Autodesk Fusion 360 part; units mm, degrees
(part 3 of 4)
sketch "Sketch28" plane through (0, 0, 0.5) normal (0, 0, 1) x (-1, 0, 0)
  circle A0 centre (52.75, -70) radius 2
  circle A1 centre (59.75, -70) radius 2
  circle A2 centre (45.75, -70) radius 2
  circle A3 centre (66.75, -70) radius 2
  circle A4 centre (38.75, -70) radius 2
  circle A5 centre (-106, -68.6442) radius 1.5
  circle A6 centre (-99, -68.6442) radius 1.5
  circle A7 centre (-92, -68.6442) radius 1.5
  circle A8 centre (-96.9706, 17.0711) radius 4.5
  line L0 (-64.4557, -59.7611) -> (-70.6729, -68.3891)
  line L1 (-70.6729, -68.3891) -> (-87.8309, -68.3891)
  line L2 (-87.8309, -68.3891) -> (-87.8309, -48.5956)
  line L3 (-87.8309, -48.5956) -> (-64.4557, -59.7611)
  line L4 (-5, -35.2698) -> (-5.0893, -45.8041)
  line L5 (-5.0893, -45.8041) -> (-79.6826, -45.1714)
  line L6 (-79.6826, -45.1714) -> (-64.4557, -34.7655)
  line L7 (-64.4557, -34.7655) -> (-5, -35.2698)
  line L8 (35, -50.5455) -> (35, -5)
  line L9 (35, -5) -> (80, 5)
  line L10 (80, 5) -> (99.8546, 5)
  line L11 (99.8546, 5) -> (35, -50.5455)
  line L12 (-49.2268, -20.3093) -> (-41.9977, -4.5677)
  line L13 (-41.9977, -4.5677) -> (-17.7598, -4.7733)
  line L14 (-17.7598, -4.7733) -> (-5, -9.2623)
  line L15 (-5, -9.2623) -> (-5.0969, -20.6836)
  line L16 (-5.0969, -20.6836) -> (-49.2268, -20.3093)
  line L17 (115, -15.9161) -> (115, -61.1347)
  line L18 (115, -61.1347) -> (67.4273, -61.1347)
  line L19 (67.4273, -61.1347) -> (115, -15.9161)
  circle A9 centre (-183, -68.6442) radius 1.5
  circle A10 centre (-155, -68.6442) radius 1.5
  circle A11 centre (-127, -68.6442) radius 1.5
  circle A12 centre (-120, -68.6442) radius 1.5
  circle A13 centre (-148, -68.6442) radius 1.5
  circle A14 centre (-176, -68.6442) radius 1.5
  circle A15 centre (-162, -68.6442) radius 1.5
  circle A16 centre (-134, -68.6442) radius 1.5
  circle A17 centre (-113, -68.6442) radius 1.5
  circle A18 centre (-141, -68.6442) radius 1.5
  circle A19 centre (-169, -68.6442) radius 1.5
  circle A20 centre (-181.8234, 101.9239) radius 4.5
  circle A21 centre (-125.2548, 45.3553) radius 4.5
  circle A22 centre (-139.397, 59.4975) radius 4.5
  circle A23 centre (-167.6812, 87.7817) radius 4.5
  circle A24 centre (-111.1127, 31.2132) radius 4.5
  circle A25 centre (-153.5391, 73.6396) radius 4.5
  circle A26 centre (87.75, -70) radius 2
  circle A27 centre (108.75, -70) radius 2
  circle A28 centre (80.75, -70) radius 2
  circle A29 centre (94.75, -70) radius 2
  circle A30 centre (101.75, -70) radius 2
  circle A31 centre (73.75, -70) radius 2
  circle A32 centre (101.6789, -8.3211) radius 5
  circle A33 centre (108.75, -80) radius 2
  circle A34 centre (86.25, -80) radius 2
  circle A35 centre (63.75, -80) radius 2
  circle A36 centre (41.25, -77.5) radius 2
  circle A37 centre (73.3947, -36.6053) radius 5
  circle A38 centre (87.5368, -22.4632) radius 5
  line L20 (120, -80) -> (120, 10)
  line L21 (120, 10) -> (75, 10)
  line L22 (75, 10) -> (30, 0)
  line L23 (30, 0) -> (0, 0)
  line L24 (0, 0) -> (-45, 10)
  line L25 (-45, 10) -> (-75.7574, 10)
  line L26 (-75.7574, 10) -> (-181.8234, 116.066)
  line L27 (-181.8234, 116.066) -> (-195.9655, 101.9239)
  line L28 (-195.9655, 101.9239) -> (-90, -4.0416)
  line L29 (-90, -4.0416) -> (-90, -62.2885)
  line L30 (-90, -62.2885) -> (-190, -62.2885)
  line L31 (-190, -62.2885) -> (-190, -75)
  line L32 (-190, -75) -> (-90, -75)
  line L33 (-90, -75) -> (-90, -80)
  line L34 (-90, -80) -> (-22.5, -80)
  line L35 (-22.5, -80) -> (0, -75)
  line L36 (0, -75) -> (30, -75)
  line L37 (30, -75) -> (37.3453, -76.6323)
  line L38 (37.3453, -76.6323) -> (37.3453, -83.3677)
  line L39 (37.3453, -83.3677) -> (45.1547, -83.3677)
  line L40 (45.1547, -83.3677) -> (45.1547, -78.3677)
  line L41 (45.1547, -78.3677) -> (52.5, -80)
  line L42 (52.5, -80) -> (59.75, -80)
  line L43 (59.75, -80) -> (59.75, -85)
  line L44 (59.75, -85) -> (67.75, -85)
  line L45 (67.75, -85) -> (67.75, -80)
  line L46 (67.75, -80) -> (82.25, -80)
  line L47 (82.25, -80) -> (82.25, -85)
  line L48 (82.25, -85) -> (90.25, -85)
  line L49 (90.25, -85) -> (90.25, -80)
  line L50 (90.25, -80) -> (104.75, -80)
  line L51 (104.75, -80) -> (104.75, -85)
  line L52 (104.75, -85) -> (112.75, -85)
  line L53 (112.75, -85) -> (112.75, -80)
  line L54 (112.75, -80) -> (120, -80)
  line L55 (-14.25, -68.5) -> (-8.25, -68.5)
  line L56 (-8.25, -68.5) -> (-8.25, -71.5)
  line L57 (-8.25, -71.5) -> (-14.25, -71.5)
  line L58 (-14.25, -71.5) -> (-14.25, -68.5)
  line L59 (-72.1594, -47.0213) -> (-67.271, -50.5004)
  line L60 (-67.271, -50.5004) -> (-69.0348, -52.9787)
  line L61 (-69.0348, -52.9787) -> (-73.9232, -49.4996)
  line L62 (-73.9232, -49.4996) -> (-72.1594, -47.0213)
  line L63 (-58.1594, -27.0213) -> (-53.271, -30.5004)
  line L64 (-53.271, -30.5004) -> (-55.0348, -32.9787)
  line L65 (-55.0348, -32.9787) -> (-59.9232, -29.4996)
  line L66 (-59.9232, -29.4996) -> (-58.1594, -27.0213)
  line L67 (-10.5728, -3.1023) -> (-4.573, -3.1532)
  line L68 (-4.573, -3.1532) -> (-4.5984, -6.1531)
  line L69 (-4.5984, -6.1531) -> (-10.5982, -6.1022)
  line L70 (-10.5982, -6.1022) -> (-10.5728, -3.1023)
  line L71 (-67.8203, 7.9003) -> (-65.8203, 7.9003)
  line L72 (-65.8203, 7.9003) -> (-65.8203, 5.9003)
  line L73 (-65.8203, 5.9003) -> (-67.8203, 5.9003)
  line L74 (-67.8203, 5.9003) -> (-67.8203, 7.9003)
  line L75 (-76.9306, -16.181) -> (-75.5164, -17.5952)
  line L76 (-75.5164, -17.5952) -> (-76.9306, -19.0095)
  line L77 (-76.9306, -19.0095) -> (-78.3448, -17.5952)
  line L78 (-78.3448, -17.5952) -> (-76.9306, -16.181)
  line L79 (-87.8309, -27.9541) -> (-85.8309, -27.9541)
  line L80 (-85.8309, -27.9541) -> (-85.8309, -29.9541)
  line L81 (-85.8309, -29.9541) -> (-87.8309, -29.9541)
  line L82 (-87.8309, -29.9541) -> (-87.8309, -27.9541)
  line L83 (-66.3319, -10.7541) -> (-65.4866, -8.9415)
  line L84 (-65.4866, -8.9415) -> (-63.674, -9.7867)
  line L85 (-63.674, -9.7867) -> (-64.5193, -11.5994)
  line L86 (-64.5193, -11.5994) -> (-66.3319, -10.7541)
  line L87 (-42.179, 1.1199) -> (-36.1792, 1.0739)
  line L88 (-36.1792, 1.0739) -> (-36.2025, -1.9678)
  line L89 (-36.2025, -1.9678) -> (-42.2023, -1.9219)
  line L90 (-42.2023, -1.9219) -> (-42.179, 1.1199)
  line L91 (-10.5728, -25.1023) -> (-4.573, -25.1532)
  line L92 (-4.573, -25.1532) -> (-4.5984, -28.1531)
  line L93 (-4.5984, -28.1531) -> (-10.5982, -28.1022)
  line L94 (-10.5982, -28.1022) -> (-10.5728, -25.1023)
  line L95 (-11.9719, -47.9791) -> (-6.0721, -49.071)
  line L96 (-6.0721, -49.071) -> (-6.6181, -52.0209)
  line L97 (-6.6181, -52.0209) -> (-12.5179, -50.929)
  line L98 (-12.5179, -50.929) -> (-11.9719, -47.9791)
  line L99 (-81.75, -71.5367) -> (-75.75, -71.5367)
  line L100 (-75.75, -71.5367) -> (-75.75, -74.5367)
  line L101 (-75.75, -74.5367) -> (-81.75, -74.5367)
  line L102 (-81.75, -74.5367) -> (-81.75, -71.5367)
  line L103 (-36.75, -71.5367) -> (-30.75, -71.5367)
  line L104 (-30.75, -71.5367) -> (-30.75, -74.5367)
  line L105 (-30.75, -74.5367) -> (-36.75, -74.5367)
  line L106 (-36.75, -74.5367) -> (-36.75, -71.5367)
  line L107 (-50.7607, -47.5524) -> (-45.1333, -49.6339)
  line L108 (-45.1333, -49.6339) -> (-46.174, -52.4476)
  line L109 (-46.174, -52.4476) -> (-51.8014, -50.3661)
  line L110 (-51.8014, -50.3661) -> (-50.7607, -47.5524)
  line L111 (-43.7607, -25.5524) -> (-38.1333, -27.6339)
  line L112 (-38.1333, -27.6339) -> (-39.174, -30.4476)
  line L113 (-39.174, -30.4476) -> (-44.8014, -28.3661)
  line L114 (-44.8014, -28.3661) -> (-43.7607, -25.5524)
  line L115 (-24.686, 0.859) -> (-18.6861, 0.8794)
  line L116 (-18.6861, 0.8794) -> (-18.6759, -2.1206)
  line L117 (-18.6759, -2.1206) -> (-24.6759, -2.141)
  line L118 (-24.6759, -2.141) -> (-24.686, 0.859)
  line L119 (-62.1634, 5.9003) -> (-62.1634, 7.9003)
  line L120 (-62.1634, 7.9003) -> (-60.1634, 7.9003)
  line L121 (-60.1634, 7.9003) -> (-60.1634, 5.9003)
  line L122 (-60.1634, 5.9003) -> (-62.1634, 5.9003)
  line L123 (-72.9306, -20.181) -> (-71.5164, -21.5952)
  line L124 (-71.5164, -21.5952) -> (-72.9306, -23.0095)
  line L125 (-72.9306, -23.0095) -> (-74.3448, -21.5952)
  line L126 (-74.3448, -21.5952) -> (-72.9306, -20.181)
  line L127 (-87.8309, -19.8881) -> (-85.8309, -19.8881)
  line L128 (-85.8309, -19.8881) -> (-85.8309, -21.8881)
  line L129 (-85.8309, -21.8881) -> (-87.8309, -21.8881)
  line L130 (-87.8309, -21.8881) -> (-87.8309, -19.8881)
  line L131 (-70.6135, -6.5508) -> (-68.8009, -7.396)
  line L132 (-68.8009, -7.396) -> (-69.6461, -9.2087)
  line L133 (-69.6461, -9.2087) -> (-71.4587, -8.3634)
  line L134 (-71.4587, -8.3634) -> (-70.6135, -6.5508)
  line L135 (-35.0324, 0.9507) -> (-29.0325, 0.9195)
  line L136 (-29.0325, 0.9195) -> (-29.0481, -2.0804)
  line L137 (-29.0481, -2.0804) -> (-35.048, -2.0492)
  line L138 (-35.048, -2.0492) -> (-35.0324, 0.9507)
  line L139 (-28.0908, -25.011) -> (-22.1784, -26.0328)
  line L140 (-22.1784, -26.0328) -> (-22.6893, -28.989)
  line L141 (-22.6893, -28.989) -> (-28.6017, -27.9672)
  line L142 (-28.6017, -27.9672) -> (-28.0908, -25.011)
  line L143 (-26.6893, -51.989) -> (-32.6017, -50.9672)
  line L144 (-32.6017, -50.9672) -> (-32.0908, -48.011)
  line L145 (-32.0908, -48.011) -> (-26.1784, -49.0328)
  line L146 (-26.1784, -49.0328) -> (-26.6893, -51.989)
  line L147 (-59.25, -71.5367) -> (-53.25, -71.5367)
  line L148 (-53.25, -71.5367) -> (-53.25, -74.5367)
  line L149 (-53.25, -74.5367) -> (-59.25, -74.5367)
  line L150 (-59.25, -74.5367) -> (-59.25, -71.5367)
  line L151 (-45, -57) -> (-5, -57)
  line L152 (-5, -57) -> (-5, -60)
  line L153 (-5, -60) -> (-45, -60)
  arc A39 (-45, -60) -> (-66.3234, -75) centre (-45, -82.6562) ccw
  line L154 (-66.3234, -75) -> (-69.4872, -75)
  arc A40 (-45, -57) -> (-69.4872, -75) centre (-45, -82.6562) ccw
  line L155 (0, -5) -> (30, -5)
  line L156 (30, -5) -> (30, -70)
  line L157 (30, -70) -> (0, -70)
  line L158 (0, -70) -> (0, -5)
  arc A41 (-87.8309, -44.505) -> (-40.6089, 7.444) centre (-128.4491, 39.8542) ccw
  line L159 (-87.8309, -44.505) -> (-87.8309, -38.9188)
  arc A42 (-87.8309, -38.9188) -> (-45.6219, 8.3158) centre (-128.4491, 39.8542) ccw
  line L160 (-45.6219, 8.3158) -> (-40.6089, 7.444)
  line L161 (30, -75) -> (28, -75)
  line L162 (28, -75) -> (28, 0)
  line L163 (28, 0) -> (30, 0)
  line L164 (30, 0) -> (30, -75)
  dimension "d570" = 2
  constraint horizontal L161
  constraint vertical L162
  constraint horizontal L163
  constraint vertical L164
  constraint coincident L23 L162.end
  constraint coincident L36.end L37.start
  measures "d570" distance of L36.end L161.end
extrude "Extrude27" cut sketch "Sketch28" against normal blind 13 contours L23 L155 L162 L163 L164 | L36 L157 L161 L162 L164 bodies 1 makes body 2 at (24.1667, 66.6667, 0)
move_body "Move1" bodies 2 to x (1, 0, 0) y (0, 1, 0) z (0, 0, 1) at (80, 0, 0)
sketch "Sketch29" plane through (0, 0, 0.5) normal (0, 0, 1) x (-1, 0, 0)
  arc A0 (-167.8309, -44.505) -> (-120.6089, 7.444) centre (-208.4491, 39.8542) ccw
  line L0 (-167.8309, -44.505) -> (-167.8309, -38.9188)
  arc A1 (-167.8309, -38.9188) -> (-125.6219, 8.3158) centre (-208.4491, 39.8542) ccw
  line L1 (-125.6219, 8.3158) -> (-120.6089, 7.444)
  line L2 (-125, -57) -> (-85, -57)
  line L3 (-85, -57) -> (-85, -60)
  line L4 (-85, -60) -> (-125, -60)
  arc A2 (-125, -60) -> (-146.3234, -75) centre (-125, -82.6562) ccw
  line L5 (-146.3234, -75) -> (-149.4872, -75)
  arc A3 (-125, -57) -> (-149.4872, -75) centre (-125, -82.6562) ccw
  line L6 (-139.25, -71.5367) -> (-133.25, -71.5367)
  line L7 (-133.25, -71.5367) -> (-133.25, -74.5367)
  line L8 (-133.25, -74.5367) -> (-139.25, -74.5367)
  line L9 (-139.25, -74.5367) -> (-139.25, -71.5367)
  line L10 (-106.6893, -51.989) -> (-112.6017, -50.9672)
  line L11 (-112.6017, -50.9672) -> (-112.0908, -48.011)
  line L12 (-112.0908, -48.011) -> (-106.1784, -49.0328)
  line L13 (-106.1784, -49.0328) -> (-106.6893, -51.989)
  line L14 (-108.0908, -25.011) -> (-102.1784, -26.0328)
  line L15 (-102.1784, -26.0328) -> (-102.6893, -28.989)
  line L16 (-102.6893, -28.989) -> (-108.6017, -27.9672)
  line L17 (-108.6017, -27.9672) -> (-108.0908, -25.011)
  line L18 (-115.0324, 0.9507) -> (-109.0325, 0.9195)
  line L19 (-109.0325, 0.9195) -> (-109.0481, -2.0804)
  line L20 (-109.0481, -2.0804) -> (-115.048, -2.0492)
  line L21 (-115.048, -2.0492) -> (-115.0324, 0.9507)
  line L22 (-150.6135, -6.5508) -> (-148.8009, -7.396)
  line L23 (-148.8009, -7.396) -> (-149.6461, -9.2087)
  line L24 (-149.6461, -9.2087) -> (-151.4587, -8.3634)
  line L25 (-151.4587, -8.3634) -> (-150.6135, -6.5508)
  line L26 (-167.8309, -19.8881) -> (-165.8309, -19.8881)
  line L27 (-165.8309, -19.8881) -> (-165.8309, -21.8881)
  line L28 (-165.8309, -21.8881) -> (-167.8309, -21.8881)
  line L29 (-167.8309, -21.8881) -> (-167.8309, -19.8881)
  line L30 (-152.9306, -20.181) -> (-151.5164, -21.5952)
  line L31 (-151.5164, -21.5952) -> (-152.9306, -23.0095)
  line L32 (-152.9306, -23.0095) -> (-154.3448, -21.5952)
  line L33 (-154.3448, -21.5952) -> (-152.9306, -20.181)
  line L34 (-142.1634, 5.9003) -> (-142.1634, 7.9003)
  line L35 (-142.1634, 7.9003) -> (-140.1634, 7.9003)
  line L36 (-140.1634, 7.9003) -> (-140.1634, 5.9003)
  line L37 (-140.1634, 5.9003) -> (-142.1634, 5.9003)
  line L38 (-104.686, 0.859) -> (-98.6861, 0.8794)
  line L39 (-98.6861, 0.8794) -> (-98.6759, -2.1206)
  line L40 (-98.6759, -2.1206) -> (-104.6759, -2.141)
  line L41 (-104.6759, -2.141) -> (-104.686, 0.859)
  line L42 (-123.7607, -25.5524) -> (-118.1333, -27.6339)
  line L43 (-118.1333, -27.6339) -> (-119.174, -30.4476)
  line L44 (-119.174, -30.4476) -> (-124.8014, -28.3661)
  line L45 (-124.8014, -28.3661) -> (-123.7607, -25.5524)
  line L46 (-130.7607, -47.5524) -> (-125.1333, -49.6339)
  line L47 (-125.1333, -49.6339) -> (-126.174, -52.4476)
  line L48 (-126.174, -52.4476) -> (-131.8014, -50.3661)
  line L49 (-131.8014, -50.3661) -> (-130.7607, -47.5524)
  line L50 (-116.75, -71.5367) -> (-110.75, -71.5367)
  line L51 (-110.75, -71.5367) -> (-110.75, -74.5367)
  line L52 (-110.75, -74.5367) -> (-116.75, -74.5367)
  line L53 (-116.75, -74.5367) -> (-116.75, -71.5367)
  line L54 (-161.75, -71.5367) -> (-155.75, -71.5367)
  line L55 (-155.75, -71.5367) -> (-155.75, -74.5367)
  line L56 (-155.75, -74.5367) -> (-161.75, -74.5367)
  line L57 (-161.75, -74.5367) -> (-161.75, -71.5367)
  line L58 (-91.9719, -47.9791) -> (-86.0721, -49.071)
  line L59 (-86.0721, -49.071) -> (-86.6181, -52.0209)
  line L60 (-86.6181, -52.0209) -> (-92.5179, -50.929)
  line L61 (-92.5179, -50.929) -> (-91.9719, -47.9791)
  line L62 (-90.5728, -25.1023) -> (-84.573, -25.1532)
  line L63 (-84.573, -25.1532) -> (-84.5984, -28.1531)
  line L64 (-84.5984, -28.1531) -> (-90.5982, -28.1022)
  line L65 (-90.5982, -28.1022) -> (-90.5728, -25.1023)
  line L66 (-122.179, 1.1199) -> (-116.1792, 1.0739)
  line L67 (-116.1792, 1.0739) -> (-116.2025, -1.9678)
  line L68 (-116.2025, -1.9678) -> (-122.2023, -1.9219)
  line L69 (-122.2023, -1.9219) -> (-122.179, 1.1199)
  line L70 (-146.3319, -10.7541) -> (-145.4866, -8.9415)
  line L71 (-145.4866, -8.9415) -> (-143.674, -9.7867)
  line L72 (-143.674, -9.7867) -> (-144.5193, -11.5994)
  line L73 (-144.5193, -11.5994) -> (-146.3319, -10.7541)
  line L74 (-167.8309, -27.9541) -> (-165.8309, -27.9541)
  line L75 (-165.8309, -27.9541) -> (-165.8309, -29.9541)
  line L76 (-165.8309, -29.9541) -> (-167.8309, -29.9541)
  line L77 (-167.8309, -29.9541) -> (-167.8309, -27.9541)
  line L78 (-156.9306, -16.181) -> (-155.5164, -17.5952)
  line L79 (-155.5164, -17.5952) -> (-156.9306, -19.0095)
  line L80 (-156.9306, -19.0095) -> (-158.3448, -17.5952)
  line L81 (-158.3448, -17.5952) -> (-156.9306, -16.181)
  line L82 (-147.8203, 7.9003) -> (-145.8203, 7.9003)
  line L83 (-145.8203, 7.9003) -> (-145.8203, 5.9003)
  line L84 (-145.8203, 5.9003) -> (-147.8203, 5.9003)
  line L85 (-147.8203, 5.9003) -> (-147.8203, 7.9003)
  line L86 (-90.5728, -3.1023) -> (-84.573, -3.1532)
  line L87 (-84.573, -3.1532) -> (-84.5984, -6.1531)
  line L88 (-84.5984, -6.1531) -> (-90.5982, -6.1022)
  line L89 (-90.5982, -6.1022) -> (-90.5728, -3.1023)
  line L90 (-138.1594, -27.0213) -> (-133.271, -30.5004)
  line L91 (-133.271, -30.5004) -> (-135.0348, -32.9787)
  line L92 (-135.0348, -32.9787) -> (-139.9232, -29.4996)
  line L93 (-139.9232, -29.4996) -> (-138.1594, -27.0213)
  line L94 (-152.1594, -47.0213) -> (-147.271, -50.5004)
  line L95 (-147.271, -50.5004) -> (-149.0348, -52.9787)
  line L96 (-149.0348, -52.9787) -> (-153.9232, -49.4996)
  line L97 (-153.9232, -49.4996) -> (-152.1594, -47.0213)
  line L98 (-94.25, -68.5) -> (-88.25, -68.5)
  line L99 (-88.25, -68.5) -> (-88.25, -71.5)
  line L100 (-88.25, -71.5) -> (-94.25, -71.5)
  line L101 (-94.25, -71.5) -> (-94.25, -68.5)
  circle A4 centre (-233.5391, 73.6396) radius 4.5
  circle A5 centre (-191.1127, 31.2132) radius 4.5
  circle A6 centre (-247.6812, 87.7817) radius 4.5
  circle A7 centre (-219.397, 59.4975) radius 4.5
  circle A8 centre (-205.2548, 45.3553) radius 4.5
  circle A9 centre (-261.8234, 101.9239) radius 4.5
  circle A10 centre (-249, -68.6442) radius 1.5
  circle A11 centre (-221, -68.6442) radius 1.5
  circle A12 centre (-193, -68.6442) radius 1.5
  circle A13 centre (-214, -68.6442) radius 1.5
  circle A14 centre (-242, -68.6442) radius 1.5
  circle A15 centre (-256, -68.6442) radius 1.5
  circle A16 centre (-228, -68.6442) radius 1.5
  circle A17 centre (-200, -68.6442) radius 1.5
  circle A18 centre (-207, -68.6442) radius 1.5
  circle A19 centre (-235, -68.6442) radius 1.5
  circle A20 centre (-263, -68.6442) radius 1.5
  line L102 (-129.2268, -20.3093) -> (-121.9977, -4.5677)
  line L103 (-121.9977, -4.5677) -> (-97.7598, -4.7733)
  line L104 (-97.7598, -4.7733) -> (-85, -9.2623)
  line L105 (-85, -9.2623) -> (-85.0969, -20.6836)
  line L106 (-85.0969, -20.6836) -> (-129.2268, -20.3093)
  line L107 (-85, -35.2698) -> (-85.0893, -45.8041)
  line L108 (-85.0893, -45.8041) -> (-159.6826, -45.1714)
  line L109 (-159.6826, -45.1714) -> (-144.4557, -34.7655)
  line L110 (-144.4557, -34.7655) -> (-85, -35.2698)
  line L111 (-144.4557, -59.7611) -> (-150.6729, -68.3891)
  line L112 (-150.6729, -68.3891) -> (-167.8309, -68.3891)
  line L113 (-167.8309, -68.3891) -> (-167.8309, -48.5956)
  line L114 (-167.8309, -48.5956) -> (-144.4557, -59.7611)
  circle A21 centre (-176.9706, 17.0711) radius 4.5
  circle A22 centre (-172, -68.6442) radius 1.5
  circle A23 centre (-179, -68.6442) radius 1.5
  circle A24 centre (-186, -68.6442) radius 1.5
  line L115 (-52, -75) -> (-52, -70)
  line L116 (-52, -70) -> (-80, -70)
  line L117 (-80, -70) -> (-80, -5)
  line L118 (-80, -5) -> (-52, -5)
  line L119 (-52, -5) -> (-52, 0)
  line L120 (-52, 0) -> (-80, 0)
  line L121 (-80, 0) -> (-125, 10)
  line L122 (-125, 10) -> (-155.7574, 10)
  line L123 (-155.7574, 10) -> (-261.8234, 116.066)
  line L124 (-261.8234, 116.066) -> (-275.9655, 101.9239)
  line L125 (-275.9655, 101.9239) -> (-170, -4.0416)
  line L126 (-170, -4.0416) -> (-170, -62.2885)
  line L127 (-170, -62.2885) -> (-270, -62.2885)
  line L128 (-270, -62.2885) -> (-270, -75)
  line L129 (-270, -75) -> (-170, -75)
  line L130 (-170, -75) -> (-170, -80)
  line L131 (-170, -80) -> (-102.5, -80)
  line L132 (-102.5, -80) -> (-80, -75)
  line L133 (-80, -75) -> (-52, -75)
  line L134 (-80, -75) -> (-10, -75)
  line L135 (-10, -75) -> (-10, -61.9841)
  line L136 (-10, -61.9841) -> (-80, -61.9841)
  line L137 (-80, -61.9841) -> (-80, -75)
  line L138 (-80, 0) -> (-10, 0)
  line L139 (-10, 0) -> (-10, -13.016)
  line L140 (-10, -13.016) -> (-80, -13.016)
  line L141 (-80, -13.016) -> (-80, 0)
  circle A25 centre (-78, -68.4921) radius 2
  line L142 (-80, -68.4921) -> (-10, -68.4921) construction
  circle A26 centre (-74.5, -68.4921) radius 1.5 construction
  circle A27 centre (-71, -68.4921) radius 2
  circle A28 centre (-67.5, -68.4921) radius 1.5
  circle A29 centre (-64, -68.4921) radius 2
  circle A30 centre (-60.5, -68.4921) radius 1.5
  circle A31 centre (-57, -68.4921) radius 2
  circle A32 centre (-53.5, -68.4921) radius 1.5
  circle A33 centre (-50, -68.4921) radius 2
  circle A34 centre (-46.5, -68.4921) radius 1.5
  circle A35 centre (-43, -68.4921) radius 2
  circle A36 centre (-39.5, -68.4921) radius 1.5
  circle A37 centre (-36, -68.4921) radius 2
  circle A38 centre (-32.5, -68.4921) radius 1.5
  circle A39 centre (-29, -68.4921) radius 2
  circle A40 centre (-25.5, -68.4921) radius 1.5
  circle A41 centre (-22, -68.4921) radius 2
  circle A42 centre (-18.5, -68.4921) radius 1.5
  circle A43 centre (-15, -68.4921) radius 2
  line L143 (-80, -6.508) -> (-10, -6.508) construction
  circle A44 centre (-78, -6.508) radius 2
  circle A45 centre (-74.5, -6.508) radius 1.5
  circle A46 centre (-71, -6.508) radius 2
  circle A47 centre (-67.5, -6.508) radius 1.5
  circle A48 centre (-64, -6.508) radius 2
  circle A49 centre (-60.5, -6.508) radius 1.5
  circle A50 centre (-57, -6.508) radius 2
  circle A51 centre (-53.5, -6.508) radius 1.5
  circle A52 centre (-50, -6.508) radius 2
  circle A53 centre (-46.5, -6.508) radius 1.5
  circle A54 centre (-43, -6.508) radius 2
  circle A55 centre (-39.5, -6.508) radius 1.5
  circle A56 centre (-36, -6.508) radius 2
  circle A57 centre (-32.5, -6.508) radius 1.5
  circle A58 centre (-29, -6.508) radius 2
  circle A59 centre (-25.5, -6.508) radius 1.5
  circle A60 centre (-22, -6.508) radius 2
  circle A61 centre (-18.5, -6.508) radius 1.5
  circle A62 centre (-15, -6.508) radius 2
  dimension "d573" = 70
  dimension "d574" = 70
  dimension "d575" = 13.016
  dimension "d576" = 4
  dimension "d577" = 3
  dimension "d578" = 4
  dimension "d579" = 3
  dimension "d580" = 4
  dimension "d581" = 3
  dimension "d582" = 4
  dimension "d583" = 3
  dimension "d584" = 4
  dimension "d585" = 3
  dimension "d586" = 4
  dimension "d587" = 3
  dimension "d588" = 4
  dimension "d589" = 3
  dimension "d590" = 4
  dimension "d591" = 3
  dimension "d592" = 4
  dimension "d593" = 3
  dimension "d594" = 4
  dimension "d595" = 4
  dimension "d596" = 3
  dimension "d597" = 4
  dimension "d598" = 3
  dimension "d599" = 4
  dimension "d600" = 3
  dimension "d601" = 4
  dimension "d602" = 3
  dimension "d603" = 4
  dimension "d604" = 3
  dimension "d605" = 4
  dimension "d606" = 3
  dimension "d607" = 4
  dimension "d608" = 3
  dimension "d609" = 4
  dimension "d610" = 3
  dimension "d611" = 4
  dimension "d612" = 3
  dimension "d613" = 4
  constraint horizontal L134
  constraint vertical L135
  constraint horizontal L136
  constraint vertical L137
  constraint coincident L132.end L133.start
  constraint horizontal L138
  constraint vertical L139
  constraint horizontal L140
  constraint vertical L141
  constraint coincident L120.end L121.start
  constraint midpoint L137 L142.start
  constraint midpoint L135 L142.end
  constraint midpoint L141 L143.start
  constraint midpoint L139 L143.end
  constraint coincident L143.start A44
  measures "d573" distance of L132.end L134.end
  measures "d574" distance of L120.end L138.end
  measures "d575" distance of L120.end L140.end
  measures "d576" diameter of A25
  measures "d577" diameter of A26
  measures "d578" diameter of A27
  measures "d579" diameter of A28
  measures "d580" diameter of A29
  measures "d581" diameter of A30
  measures "d582" diameter of A31
  measures "d583" diameter of A32
  measures "d584" diameter of A33
  measures "d585" diameter of A34
  measures "d586" diameter of A35
  measures "d587" diameter of A36
  measures "d588" diameter of A37
  measures "d589" diameter of A38
  measures "d590" diameter of A39
  measures "d591" diameter of A40
  measures "d592" diameter of A41
  measures "d593" diameter of A42
  measures "d594" diameter of A43
  measures "d595" diameter of A44
  measures "d596" diameter of A45
  measures "d597" diameter of A46
  measures "d598" diameter of A47
  measures "d599" diameter of A48
  measures "d600" diameter of A49
  measures "d601" diameter of A50
  measures "d602" diameter of A51
  measures "d603" diameter of A52
  measures "d604" diameter of A53
  measures "d605" diameter of A54
  measures "d606" diameter of A55
  measures "d607" diameter of A56
  measures "d608" diameter of A57
  measures "d609" diameter of A58
  measures "d610" diameter of A59
  measures "d611" diameter of A60
  measures "d612" diameter of A61
  measures "d613" diameter of A62
extrude "Extrude28" add sketch "Sketch29" against normal blind 0.5 contours A43 | A41 | A39 | A37 | A33 | L115 L116 L117 L134 L135 L136 L137 A25 A27 A28 A29 A30 A31 | L116 A31 | L116 L117 L137 A25 | L116 A29 A30 A31 | L116 A25 | L116 A29 | L116 A27 A28 A29 | L116 A27 picked at (-56.9502, -68.8326) picked at (-77.7564, -68.8768) picked at (-64.0498, -68.8326) picked at (-70.3388, -68.8213) bodies 2
extrude "Extrude29" add sketch "Sketch29" against normal blind 0.5 contours A35 bodies 2
extrude "Extrude30" add sketch "Sketch29" against normal blind 0.5 contours A62 | A60 | A58 | A56 | A54 | A52 | L117 L118 L119 L138 L139 L140 L141 A44 A45 A46 A47 A48 A49 A50 | L117 L118 L141 A44 | L118 A44 | L118 A44 A45 A46 | L118 A46 | L118 A46 A47 A48 | L118 A48 | L118 A50 | L118 A48 A49 A50 picked at (-78.3104, -6.1905) picked at (-70.8517, -6.1526) picked at (-63.9502, -6.1675) picked at (-57.0498, -6.1675) bodies 2
sketch "Sketch30" plane through (0, 0, 0.5) normal (0, 0, 1) x (-1, 0, 0)
  line L0 (30, 0) -> (30, -75)
  line L1 (30, -75) -> (37.3453, -76.6323)
  line L2 (37.3453, -76.6323) -> (37.3453, -83.3677)
  line L3 (37.3453, -83.3677) -> (45.1547, -83.3677)
  line L4 (45.1547, -83.3677) -> (45.1547, -78.3677)
  line L5 (45.1547, -78.3677) -> (52.5, -80)
  line L6 (52.5, -80) -> (59.75, -80)
  line L7 (59.75, -80) -> (59.75, -85)
  line L8 (59.75, -85) -> (67.75, -85)
  line L9 (67.75, -85) -> (67.75, -80)
  line L10 (67.75, -80) -> (82.25, -80)
  line L11 (82.25, -80) -> (82.25, -85)
  line L12 (82.25, -85) -> (90.25, -85)
  line L13 (90.25, -85) -> (90.25, -80)
  line L14 (90.25, -80) -> (104.75, -80)
  line L15 (104.75, -80) -> (104.75, -85)
  line L16 (104.75, -85) -> (112.75, -85)
  line L17 (112.75, -85) -> (112.75, -80)
  line L18 (112.75, -80) -> (120, -80)
  line L19 (120, -80) -> (120, 10)
  line L20 (120, 10) -> (75, 10)
  line L21 (75, 10) -> (30, 0)
  circle A0 centre (52.75, -70) radius 2
  circle A1 centre (59.75, -70) radius 2
  circle A2 centre (45.75, -70) radius 2
  circle A3 centre (66.75, -70) radius 2
  circle A4 centre (38.75, -70) radius 2
  line L22 (35, -50.5455) -> (35, -5)
  line L23 (35, -5) -> (80, 5)
  line L24 (80, 5) -> (99.8546, 5)
  line L25 (99.8546, 5) -> (35, -50.5455)
  line L26 (115, -15.9161) -> (115, -61.1347)
  line L27 (115, -61.1347) -> (67.4273, -61.1347)
  line L28 (67.4273, -61.1347) -> (115, -15.9161)
  circle A5 centre (87.75, -70) radius 2
  circle A6 centre (108.75, -70) radius 2
  circle A7 centre (80.75, -70) radius 2
  circle A8 centre (94.75, -70) radius 2
  circle A9 centre (101.75, -70) radius 2
  circle A10 centre (73.75, -70) radius 2
  circle A11 centre (101.6789, -8.3211) radius 5
  circle A12 centre (108.75, -80) radius 2
  circle A13 centre (86.25, -80) radius 2
  circle A14 centre (63.75, -80) radius 2
  circle A15 centre (41.25, -77.5) radius 2
  circle A16 centre (73.3947, -36.6053) radius 5
  circle A17 centre (87.5368, -22.4632) radius 5
  line L29 (30, 0) -> (94.8932, 0)
  line L30 (94.8932, 0) -> (94.8932, -13.016)
  line L31 (94.8932, -13.016) -> (30, -13.016)
  line L32 (30, -13.016) -> (30, 0)
  line L33 (30, -6.508) -> (94.8932, -6.508) construction
  circle A18 centre (35, -6.508) radius 5 construction
  circle A19 centre (42, -6.508) radius 2
  circle A20 centre (45.5, -6.508) radius 1.5 construction
  circle A21 centre (49, -6.508) radius 2
  circle A22 centre (52.5, -6.508) radius 1.5 construction
  circle A23 centre (56, -6.508) radius 2
  circle A24 centre (59.5, -6.508) radius 1.5 construction
  circle A25 centre (63, -6.508) radius 2
  circle A26 centre (66.5, -6.508) radius 1.5 construction
  circle A27 centre (70, -6.508) radius 2
  circle A28 centre (73.5, -6.508) radius 1.5 construction
  circle A29 centre (77, -6.508) radius 2
  circle A30 centre (80.5, -6.508) radius 1.5 construction
  circle A31 centre (84, -6.508) radius 2
  circle A32 centre (42, -6.508) radius 3
  circle A33 centre (49, -6.508) radius 3
  circle A34 centre (56, -6.508) radius 3
  circle A35 centre (63, -6.508) radius 3
  circle A36 centre (70, -6.508) radius 3
  circle A37 centre (77, -6.508) radius 3
  circle A38 centre (84, -6.508) radius 3
  circle A39 centre (88.5, -6.508) radius 1.5 construction
  circle A40 centre (92, -6.508) radius 2
  circle A41 centre (95.4998, -6.5337) radius 1.5 construction
  circle A42 centre (98.9994, -6.5337) radius 2
  circle A43 centre (102.4992, -6.508) radius 1.5 construction
  circle A44 centre (105.9992, -6.508) radius 2
  circle A45 centre (109.4992, -6.508) radius 1.5 construction
  circle A46 centre (112.9992, -6.508) radius 2
  circle A47 centre (116.4992, -6.508) radius 1.5 construction
  circle A48 centre (92, -6.508) radius 3
  circle A49 centre (98.9994, -6.5337) radius 3
  circle A50 centre (105.9992, -6.508) radius 3
  circle A51 centre (112.9992, -6.508) radius 3
  dimension "d620" = 13.016
  dimension "d621" = 10
  dimension "d622" = 4
  dimension "d623" = 3
  dimension "d624" = 4
  dimension "d625" = 3
  dimension "d626" = 4
  dimension "d627" = 3
  dimension "d628" = 4
  dimension "d629" = 3
  dimension "d630" = 4
  dimension "d631" = 3
  dimension "d632" = 4
  dimension "d633" = 3
  dimension "d634" = 4
  dimension "d635" = 1
  dimension "d636" = 1
  dimension "d637" = 1
  dimension "d638" = 1
  dimension "d639" = 1
  dimension "d640" = 1
  dimension "d641" = 1
  dimension "d706" = 3
  dimension "d707" = 4
  dimension "d708" = 3
  dimension "d709" = 4
  dimension "d710" = 3
  dimension "d711" = 4
  dimension "d712" = 3
  dimension "d713" = 4
  dimension "d714" = 3
  dimension "d715" = 1
  dimension "d716" = 1
  dimension "d717" = 1
  dimension "d718" = 1
  constraint horizontal L29
  constraint vertical L30
  constraint horizontal L31
  constraint vertical L32
  constraint coincident L0.start L21.end
  constraint midpoint L32 L33.start
  constraint midpoint L30 L33.end
  constraint coincident L33.start A18
  measures "d620" distance of L0.start L31.end
  measures "d621" diameter of A18
  measures "d622" diameter of A19
  measures "d623" diameter of A20
  measures "d624" diameter of A21
  measures "d625" diameter of A22
  measures "d626" diameter of A23
  measures "d627" diameter of A24
  measures "d628" diameter of A25
  measures "d629" diameter of A26
  measures "d630" diameter of A27
  measures "d631" diameter of A28
  measures "d632" diameter of A29
  measures "d633" diameter of A30
  measures "d634" diameter of A31
  measures "d706" diameter of A39
  measures "d707" diameter of A40
  measures "d708" diameter of A41
  measures "d709" diameter of A42
  measures "d710" diameter of A43
  measures "d711" diameter of A44
  measures "d712" diameter of A45
  measures "d713" diameter of A46
  measures "d714" diameter of A47
extrude "Extrude31" add sketch "Sketch30" against normal blind 0.5 contours L22 L23 L25 L29 L31 A32 A38 | L23 A32 | L25 A31 A38 | L25 A31 | A19 | A21 | A23 | A25 | A27 | A29 | A33 | A34 | A35 | A36 | A37 picked at (41.4192, -3.9118) picked at (82.9913, -8.9706) picked at (85.1845, -6.7668) bodies 1
extrude "Extrude32" add sketch "Sketch30" along normal blind 2 contours L25 A31 | L25 A31 | A19 | A21 | A23 | A25 | A27 | A29 bodies 1
sphere "SpherePrimitive22" add diameter 5 placed x (-1, 0, 0) y (0, -1, 0) z (0, 0, 1) at (-84, 6.508, 2.5) bodies 1
sphere "SpherePrimitive23" add diameter 5 placed x (-1, 0, 0) y (0, -1, 0) z (0, 0, 1) at (-77, 6.508, 2.5) bodies 1
sphere "SpherePrimitive24" add diameter 5 placed x (-1, 0, 0) y (0, -1, 0) z (0, 0, 1) at (-70, 6.508, 2.5) bodies 1
sphere "SpherePrimitive25" add diameter 5 placed x (-1, 0, 0) y (0, -1, 0) z (0, 0, 1) at (-63, 6.508, 2.5) bodies 1
sphere "SpherePrimitive26" add diameter 5 placed x (-1, 0, 0) y (0, -1, 0) z (0, 0, 1) at (-56, 6.508, 2.5) bodies 1
sphere "SpherePrimitive27" add diameter 5 placed x (-1, 0, 0) y (0, -1, 0) z (0, 0, 1) at (-49, 6.508, 2.5) bodies 1
sphere "SpherePrimitive28" add diameter 5 placed x (-1, 0, 0) y (0, -1, 0) z (0, 0, 1) at (-42, 6.508, 2.5) bodies 1
extrude "Extrude33" cut sketch "Sketch30" along normal blind 2 contours L23 A32 | L25 A31 A38 | L25 A31 A38 | A33 | A34 | A35 | A36 | A37 picked at (41.4192, -3.9118) bodies 1
extrude "Extrude34" add 1 faces at (122.2799, -7.7346, 0.1667) along direction (0.171325, 0.985215, 0) blind 4 on bodies 2 bodies 2
extrude "Extrude35" add 1 faces at (125.8503, -7.0022, 0.1667) along direction (0.985215, -0.171325, 0) blind 2 on bodies 2 bodies 2
extrude "Extrude36" add 1 faces at (167.8309, 40.7809, 0.3333) along direction (-1, 0, 0) blind 6 on bodies 2 bodies 2
extrude "Extrude37" add 1 faces at (161.8309, 40.5352, 0.3333) along direction (-1, 0, 0) blind 4.5 on bodies 2 bodies 2
extrude "Extrude38" add 1 faces at (164.5011, 38.9188, 0.1667) along direction (0, -1, 0) blind 3.5 on bodies 2 bodies 2
extrude "Extrude39" cut 8 faces at (166.4976, 28.6208, 2) (166.4976, 20.5548, 2) (152.4592, 21.5952, 2) (156.4592, 17.5952, 2) (144.56, 10.1092, 2) (150.5728, 8.041, 2) (146.4869, -7.2336, 2) (140.8301, -7.2336, 2) along direction (0, 0, -1) blind 1.5 on bodies 2 bodies 2
sketch "Sketch38" plane through (0, 0, 0.5) normal (0, 0, 1) x (-1, 0, 0)
  circle A0 centre (-32.5, -6.508) radius 1.5
  circle A1 centre (-60.5, -6.508) radius 1.5
  circle A2 centre (-67.5, -6.508) radius 1.5
  circle A3 centre (-53.5, -6.508) radius 1.5
  circle A4 centre (-25.5, -6.508) radius 1.5
  circle A5 centre (-18.5, -6.508) radius 1.5
  circle A6 centre (-39.5, -6.508) radius 1.5
  circle A7 centre (-46.5, -6.508) radius 1.5
  circle A8 centre (-74.5, -6.508) radius 1.5
  circle A9 centre (-39.5, -68.4921) radius 1.5
  circle A10 centre (-18.5, -68.4921) radius 1.5
  circle A11 centre (-46.5, -68.4921) radius 1.5
  circle A12 centre (-32.5, -68.4921) radius 1.5
  circle A13 centre (-25.5, -68.4921) radius 1.5
  circle A14 centre (-67.5, -68.4921) radius 1.5
  circle A15 centre (-53.5, -68.4921) radius 1.5
  circle A16 centre (-60.5, -68.4921) radius 1.5
  line L0 (-125, -57) -> (-85, -57)
  line L1 (-85, -57) -> (-85, -60)
  line L2 (-85, -60) -> (-125, -60)
  arc A17 (-125, -60) -> (-146.3234, -75) centre (-125, -82.6562) ccw
  line L3 (-146.3234, -75) -> (-149.4872, -75)
  arc A18 (-125, -57) -> (-149.4872, -75) centre (-125, -82.6562) ccw
  line L4 (-139.25, -71.5367) -> (-133.25, -71.5367)
  line L5 (-133.25, -71.5367) -> (-133.25, -74.5367)
  line L6 (-133.25, -74.5367) -> (-139.25, -74.5367)
  line L7 (-139.25, -74.5367) -> (-139.25, -71.5367)
  line L8 (-106.6893, -51.989) -> (-112.6017, -50.9672)
  line L9 (-112.6017, -50.9672) -> (-112.0908, -48.011)
  line L10 (-112.0908, -48.011) -> (-106.1784, -49.0328)
  line L11 (-106.1784, -49.0328) -> (-106.6893, -51.989)
  line L12 (-108.0908, -25.011) -> (-102.1784, -26.0328)
  line L13 (-102.1784, -26.0328) -> (-102.6893, -28.989)
  line L14 (-102.6893, -28.989) -> (-108.6017, -27.9672)
  line L15 (-108.6017, -27.9672) -> (-108.0908, -25.011)
  line L16 (-115.0324, 0.9507) -> (-109.0325, 0.9195)
  line L17 (-109.0325, 0.9195) -> (-109.0481, -2.0804)
  line L18 (-109.0481, -2.0804) -> (-115.048, -2.0492)
  line L19 (-115.048, -2.0492) -> (-115.0324, 0.9507)
  line L20 (-104.686, 0.859) -> (-98.6861, 0.8794)
  line L21 (-98.6861, 0.8794) -> (-98.6759, -2.1206)
  line L22 (-98.6759, -2.1206) -> (-104.6759, -2.141)
  line L23 (-104.6759, -2.141) -> (-104.686, 0.859)
  line L24 (-123.7607, -25.5524) -> (-118.1333, -27.6339)
  line L25 (-118.1333, -27.6339) -> (-119.174, -30.4476)
  line L26 (-119.174, -30.4476) -> (-124.8014, -28.3661)
  line L27 (-124.8014, -28.3661) -> (-123.7607, -25.5524)
  line L28 (-130.7607, -47.5524) -> (-125.1333, -49.6339)
  line L29 (-125.1333, -49.6339) -> (-126.174, -52.4476)
  line L30 (-126.174, -52.4476) -> (-131.8014, -50.3661)
  line L31 (-131.8014, -50.3661) -> (-130.7607, -47.5524)
  line L32 (-116.75, -71.5367) -> (-110.75, -71.5367)
  line L33 (-110.75, -71.5367) -> (-110.75, -74.5367)
  line L34 (-110.75, -74.5367) -> (-116.75, -74.5367)
  line L35 (-116.75, -74.5367) -> (-116.75, -71.5367)
  line L36 (-161.75, -71.5367) -> (-155.75, -71.5367)
  line L37 (-155.75, -71.5367) -> (-155.75, -74.5367)
  line L38 (-155.75, -74.5367) -> (-161.75, -74.5367)
  line L39 (-161.75, -74.5367) -> (-161.75, -71.5367)
  line L40 (-91.9719, -47.9791) -> (-86.0721, -49.071)
  line L41 (-86.0721, -49.071) -> (-86.6181, -52.0209)
  line L42 (-86.6181, -52.0209) -> (-92.5179, -50.929)
  line L43 (-92.5179, -50.929) -> (-91.9719, -47.9791)
  line L44 (-90.5728, -25.1023) -> (-84.573, -25.1532)
  line L45 (-84.573, -25.1532) -> (-84.5984, -28.1531)
  line L46 (-84.5984, -28.1531) -> (-90.5982, -28.1022)
  line L47 (-90.5982, -28.1022) -> (-90.5728, -25.1023)
  line L48 (-122.179, 1.1199) -> (-116.1792, 1.0739)
  line L49 (-116.1792, 1.0739) -> (-116.2025, -1.9678)
  line L50 (-116.2025, -1.9678) -> (-122.2023, -1.9219)
  line L51 (-122.2023, -1.9219) -> (-122.179, 1.1199)
  line L52 (-90.5728, -3.1023) -> (-84.573, -3.1532)
  line L53 (-84.573, -3.1532) -> (-84.5984, -6.1531)
  line L54 (-84.5984, -6.1531) -> (-90.5982, -6.1022)
  line L55 (-90.5982, -6.1022) -> (-90.5728, -3.1023)
  line L56 (-138.1594, -27.0213) -> (-133.271, -30.5004)
  line L57 (-133.271, -30.5004) -> (-135.0348, -32.9787)
  line L58 (-135.0348, -32.9787) -> (-139.9232, -29.4996)
  line L59 (-139.9232, -29.4996) -> (-138.1594, -27.0213)
  line L60 (-152.1594, -47.0213) -> (-147.271, -50.5004)
  line L61 (-147.271, -50.5004) -> (-149.0348, -52.9787)
  line L62 (-149.0348, -52.9787) -> (-153.9232, -49.4996)
  line L63 (-153.9232, -49.4996) -> (-152.1594, -47.0213)
  line L64 (-94.25, -68.5) -> (-88.25, -68.5)
  line L65 (-88.25, -68.5) -> (-88.25, -71.5)
  line L66 (-88.25, -71.5) -> (-94.25, -71.5)
  line L67 (-94.25, -71.5) -> (-94.25, -68.5)
  circle A19 centre (-233.5391, 73.6396) radius 4.5
  circle A20 centre (-191.1127, 31.2132) radius 4.5
  circle A21 centre (-247.6812, 87.7817) radius 4.5
  circle A22 centre (-219.397, 59.4975) radius 4.5
  circle A23 centre (-205.2548, 45.3553) radius 4.5
  circle A24 centre (-261.8234, 101.9239) radius 4.5
  circle A25 centre (-249, -68.6442) radius 1.5
  circle A26 centre (-221, -68.6442) radius 1.5
  circle A27 centre (-193, -68.6442) radius 1.5
  circle A28 centre (-214, -68.6442) radius 1.5
  circle A29 centre (-242, -68.6442) radius 1.5
  circle A30 centre (-256, -68.6442) radius 1.5
  circle A31 centre (-228, -68.6442) radius 1.5
  circle A32 centre (-200, -68.6442) radius 1.5
  circle A33 centre (-207, -68.6442) radius 1.5
  circle A34 centre (-235, -68.6442) radius 1.5
  circle A35 centre (-263, -68.6442) radius 1.5
  line L68 (-129.2268, -20.3093) -> (-121.9977, -4.5677)
  line L69 (-121.9977, -4.5677) -> (-97.7598, -4.7733)
  line L70 (-97.7598, -4.7733) -> (-85, -9.2623)
  line L71 (-85, -9.2623) -> (-85.0969, -20.6836)
  line L72 (-85.0969, -20.6836) -> (-129.2268, -20.3093)
  line L73 (-85, -35.2698) -> (-85.0893, -45.8041)
  line L74 (-85.0893, -45.8041) -> (-159.6826, -45.1714)
  line L75 (-159.6826, -45.1714) -> (-144.4557, -34.7655)
  line L76 (-144.4557, -34.7655) -> (-85, -35.2698)
  line L77 (-144.4557, -59.7611) -> (-150.6729, -68.3891)
  line L78 (-150.6729, -68.3891) -> (-167.8309, -68.3891)
  line L79 (-167.8309, -68.3891) -> (-167.8309, -48.5956)
  line L80 (-167.8309, -48.5956) -> (-144.4557, -59.7611)
  circle A36 centre (-176.9706, 17.0711) radius 4.5
  circle A37 centre (-172, -68.6442) radius 1.5
  circle A38 centre (-179, -68.6442) radius 1.5
  circle A39 centre (-186, -68.6442) radius 1.5
  line L81 (-80, -75) -> (-10, -75)
  line L82 (-10, -75) -> (-10, -61.9841)
  line L83 (-10, -61.9841) -> (-80, -61.9841)
  line L84 (-80, -61.9841) -> (-80, -13.016)
  line L85 (-80, -13.016) -> (-10, -13.016)
  line L86 (-10, -13.016) -> (-10, 0)
  line L87 (-10, 0) -> (-80, 0)
  line L88 (-80, 0) -> (-125, 10)
  line L89 (-125, 10) -> (-155.7574, 10)
  line L90 (-155.7574, 10) -> (-261.8234, 116.066)
  line L91 (-261.8234, 116.066) -> (-275.9655, 101.9239)
  line L92 (-275.9655, 101.9239) -> (-170, -4.0416)
  line L93 (-170, -4.0416) -> (-170, -62.2885)
  line L94 (-170, -62.2885) -> (-270, -62.2885)
  line L95 (-270, -62.2885) -> (-270, -75)
  line L96 (-270, -75) -> (-170, -75)
  line L97 (-170, -75) -> (-170, -80)
  line L98 (-170, -80) -> (-102.5, -80)
  line L99 (-102.5, -80) -> (-80, -75)
  arc A40 (-161.6623, -35.4188) -> (-127.1667, 4.5244) centre (-208.4491, 39.8542) ccw
  line L100 (-127.1667, 4.5244) -> (-122.1059, 3.6443)
  arc A41 (-157.8415, -38.9188) -> (-122.1059, 3.6443) centre (-208.4491, 39.8542) ccw
  line L101 (-80, 0) -> (-218.5188, 0) construction
  line L102 (-155.7574, 10) -> (-170, 0) construction
  line L103 (-155.7574, 10) -> (-125, 10) construction
  line L104 (-125, 10) -> (-80, 0) construction
  line L105 (-170, 0) -> (-270, 0)
  line L106 (-270, 0) -> (-270, -13.016)
  line L107 (-270, -13.016) -> (-170, -13.016)
  line L108 (-170, -13.016) -> (-170, 0)
  line L109 (-170, -6.508) -> (-270, -6.508) construction
  circle A42 centre (-171.5, -6.508) radius 1.5
  circle A43 centre (-175, -6.508) radius 2
  circle A44 centre (-178.5, -6.508) radius 1.5
  circle A45 centre (-182, -6.508) radius 2
  circle A46 centre (-185.5, -6.508) radius 1.5
  circle A47 centre (-189, -6.508) radius 2
  circle A48 centre (-192.5, -6.508) radius 1.5
  circle A49 centre (-196, -6.508) radius 2
  circle A50 centre (-199.5, -6.508) radius 1.5
  circle A51 centre (-203, -6.508) radius 2
  circle A52 centre (-206.5, -6.508) radius 1.5
  circle A53 centre (-210, -6.508) radius 2
  circle A54 centre (-213.5, -6.508) radius 1.5
  circle A55 centre (-217, -6.508) radius 2
  circle A56 centre (-220.5, -6.508) radius 1.5
  circle A57 centre (-224, -6.508) radius 2
  circle A58 centre (-227.5, -6.508) radius 1.5
  circle A59 centre (-231, -6.508) radius 2
  circle A60 centre (-234.5, -6.508) radius 1.5
  circle A61 centre (-238.1494, -6.8294) radius 2
  circle A62 centre (-241.5, -6.508) radius 1.5
  circle A63 centre (-245, -6.508) radius 2
  circle A64 centre (-248.5, -6.508) radius 1.5
  circle A65 centre (-252, -6.508) radius 2
  circle A66 centre (-255.5, -6.508) radius 1.5
  circle A67 centre (-259, -6.508) radius 2
  circle A68 centre (-262.5, -6.508) radius 1.5
  circle A69 centre (-266, -6.508) radius 2
  line L110 (-155.7574, 10) -> (-170, 0)
  line L111 (-170, 0) -> (-173.9934, 0)
  line L112 (-173.9934, 0) -> (-275.9655, 101.9239)
  line L113 (-275.9655, 101.9239) -> (-261.8234, 116.066)
  line L114 (-261.8234, 116.066) -> (-155.7574, 10)
  line L115 (-127.1667, 4.5244) -> (-154.2321, 4.5244)
  line L116 (-161.6623, -35.4188) -> (-161.6623, 0)
  line L117 (-154.2321, 4.5244) -> (-161.6623, 0)
  arc A70 (-161.6623, -35.4188) -> (-127.1667, 4.5244) centre (-208.4491, 39.8542) ccw
  line L118 (-157.8415, -38.9188) -> (-157.8415, -35.4188)
  line L119 (-157.8415, -35.4188) -> (-161.6623, -35.4188)
  circle A71 centre (-238.1494, 8.1706) radius 2
  circle A72 centre (-241.5, 8.492) radius 1.5
  circle A73 centre (-245, 8.492) radius 2
  circle A74 centre (-248.5, 8.492) radius 1.5
  circle A75 centre (-252, 8.492) radius 2
  circle A76 centre (-255.5, 8.492) radius 1.5
  circle A77 centre (-259, 8.492) radius 2
  circle A78 centre (-262.5, 8.492) radius 1.5
  circle A79 centre (-266, 8.492) radius 2
  circle A80 centre (-234.5, 8.492) radius 1.5
  circle A81 centre (-231, 8.492) radius 2
  circle A82 centre (-227.5, 8.492) radius 1.5
  circle A83 centre (-224, 8.492) radius 2
  circle A84 centre (-220.5, 8.492) radius 1.5
  circle A85 centre (-217, 8.492) radius 2
  circle A86 centre (-206.5, 8.492) radius 1.5
  circle A87 centre (-210, 8.492) radius 2
  circle A88 centre (-213.5, 8.492) radius 1.5
  circle A89 centre (-203, 8.492) radius 2
  circle A90 centre (-199.5, 8.492) radius 1.5
  circle A91 centre (-196, 8.492) radius 2
  circle A92 centre (-192.5, 8.492) radius 1.5
  circle A93 centre (-189, 8.492) radius 2
  circle A94 centre (-185.5, 8.492) radius 1.5
  circle A95 centre (-182, 8.492) radius 2
  circle A96 centre (-178.5, 8.492) radius 1.5
  circle A97 centre (-175, 8.492) radius 2
  circle A98 centre (-171.5, 8.492) radius 1.5
  line L120 (-270, 8.492) -> (-270, 1.984)
  line L121 (-270, 8.492) -> (-270, 15)
  line L122 (-270, 1.984) -> (-123.7944, 1.984)
  line L123 (-123.7944, 1.984) -> (-123.7944, 15)
  line L124 (-123.7944, 15) -> (-270, 15)
  line L125 (-270, 15) -> (-270, 1.984)
  line L126 (-123.7944, 15) -> (-108.0327, 6.2295)
  line L127 (-108.0327, 6.2295) -> (-123.7944, 1.984)
  dimension "d669" = 13.016
  dimension "d670" = 3
  dimension "d671" = 4
  dimension "d672" = 3
  dimension "d673" = 4
  dimension "d674" = 3
  dimension "d675" = 4
  dimension "d676" = 3
  dimension "d677" = 4
  dimension "d678" = 3
  dimension "d679" = 4
  dimension "d680" = 3
  dimension "d681" = 4
  dimension "d682" = 3
  dimension "d683" = 4
  dimension "d684" = 3
  dimension "d685" = 4
  dimension "d686" = 3
  dimension "d687" = 4
  dimension "d688" = 3
  dimension "d689" = 4
  dimension "d690" = 3
  dimension "d691" = 4
  dimension "d692" = 3
  dimension "d693" = 4
  dimension "d694" = 3
  dimension "d695" = 4
  dimension "d696" = 3
  dimension "d697" = 4
  dimension "d727" = 3
  dimension "d728" = 4
  dimension "d729" = 3
  dimension "d730" = 4
  dimension "d731" = 3
  dimension "d732" = 4
  dimension "d733" = 3
  dimension "d734" = 4
  dimension "d735" = 3
  dimension "d736" = 4
  dimension "d737" = 3
  dimension "d738" = 4
  dimension "d739" = 3
  dimension "d740" = 4
  dimension "d741" = 3
  dimension "d742" = 4
  dimension "d743" = 3
  dimension "d744" = 4
  dimension "d745" = 3
  dimension "d746" = 4
  dimension "d747" = 3
  dimension "d748" = 4
  dimension "d749" = 3
  dimension "d750" = 4
  dimension "d751" = 3
  dimension "d752" = 4
  dimension "d753" = 3
  dimension "d754" = 4
  dimension "d755" = 6.508
  dimension "d756" = 6.508
  constraint horizontal L101
  constraint coincident L87.end L88.start
  constraint coincident L89.end L90.start
  constraint coincident L101 L102.end
  constraint coincident L88.end L89.start
  constraint horizontal L105
  constraint vertical L106
  constraint horizontal L107
  constraint vertical L108
  constraint midpoint L108 L109.start
  constraint midpoint L106 L109.end
  constraint coincident L109.start A42
  constraint coincident L105 L111.end
  constraint coincident L91.end L92.start
  constraint coincident L90.end L91.start
  constraint coincident A40.end L100.start
  constraint parallel L101 L115
  constraint coincident A40.start L116.start
  constraint coincident L101 L116.end
  constraint perpendicular L101 L116
  constraint horizontal L122
  constraint vertical L123
  constraint horizontal L124
  constraint vertical L125
  constraint coincident L104 L126.end
  measures "d669" distance of L102.end L107.end
  measures "d670" diameter of A42
  measures "d671" diameter of A43
  measures "d672" diameter of A44
  measures "d673" diameter of A45
  measures "d674" diameter of A46
  measures "d675" diameter of A47
  measures "d676" diameter of A48
  measures "d677" diameter of A49
  measures "d678" diameter of A50
  measures "d679" diameter of A51
  measures "d680" diameter of A52
  measures "d681" diameter of A53
  measures "d682" diameter of A54
  measures "d683" diameter of A55
  measures "d684" diameter of A56
  measures "d685" diameter of A57
  measures "d686" diameter of A58
  measures "d687" diameter of A59
  measures "d688" diameter of A60
  measures "d689" diameter of A61
  measures "d690" diameter of A62
  measures "d691" diameter of A63
  measures "d692" diameter of A64
  measures "d693" diameter of A65
  measures "d694" diameter of A66
  measures "d695" diameter of A67
  measures "d696" diameter of A68
  measures "d697" diameter of A69
  measures "d727" diameter of A98
  measures "d728" diameter of A97
  measures "d729" diameter of A96
  measures "d730" diameter of A95
  measures "d731" diameter of A94
  measures "d732" diameter of A93
  measures "d733" diameter of A92
  measures "d734" diameter of A91
  measures "d735" diameter of A90
  measures "d736" diameter of A89
  measures "d737" diameter of A86
  measures "d738" diameter of A87
  measures "d739" diameter of A88
  measures "d740" diameter of A85
  measures "d741" diameter of A84
  measures "d742" diameter of A83
  measures "d743" diameter of A82
  measures "d744" diameter of A81
  measures "d745" diameter of A80
  measures "d746" diameter of A71
  measures "d747" diameter of A72
  measures "d748" diameter of A73
  measures "d749" diameter of A74
  measures "d750" diameter of A75
  measures "d751" diameter of A76
  measures "d752" diameter of A77
  measures "d753" diameter of A78
  measures "d754" diameter of A79
  measures "d755" distance of L120.start L120.end
  measures "d756" distance of L120.start L121.end
extrude "Extrude40" cut sketch "Sketch38" against normal blind 10 contours A36 L90 L91 L112 L113 L114 L124 | A98 | A97 | A96 | A36 L90 L110 L112 L114 A95 L122 L124 | L112 A95 | L105 L110 L111 L112 L122 | A40 L116 L117 A70 L122 | A40 L115 L117 A70 L122 bodies 2
extrude "Extrude41" add sketch "Sketch38" against normal blind 0.5 contours A59 | A57 | A55 | A53 | A51 | A49 | A47 | A45 | A43 | L92 L93 L105 L106 L107 L108 | A61 A62 | A69 | A67 | A65 | A63 picked at (-237.4452, -6.8912) bodies 2